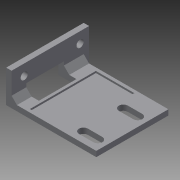
# Autodesk Inventor part: bart z endstop bracket v9
Saved by Autodesk Inventor 2014 SP1 (Build 180222100, 222)
## iProperties
Created: 2015-07-08
Part Number: bart z endstop bracket v9
Material: Generic
Document SubType Name: Modeling
Designer: Mon
Density: 1 g/cm^3
Appearance: Default
Author: Mon
Autodesk Inventor part; units mm, degrees
ref_plane "YZ Plane" through (0, 0, 0) normal (1, 0, 0) x (0, 1, 0)
ref_plane "XZ Plane" through (0, 0, 0) normal (0, 1, 0) x (-1, 0, 0)
ref_plane "XY Plane" through (0, 0, 0) normal (0, 0, 1) x (1, 0, 0)
sketch "Sketch1" plane through (0, 0, 0) normal (0, 0, 1) x (1, 0, 0)
  line L0 (0, 0) -> (50, 0)
  line L1 (50, 0) -> (50, -40)
  line L2 (50, -40) -> (0, -40)
  line L3 (0, -40) -> (0, 0)
  dimension "d0" = 50
  dimension "d1" = 40
  constraints: 8 end point, 2 parallel, 1 horizontal, 1 perpendicular
  measures "d0" distance of L1.end L2.end
  measures "d1" distance of L0.end L1.end
extrude "Extrusion1" add sketch "Sketch1" along normal blind 3
sketch "Sketch2" plane through (0, 0, 3) normal (0, 0, 1) x (1, 0, 0)
  line L0 (0, -40) -> (50, -40) projected
  line L1 (0, 0) -> (3, 0)
  line L2 (3, 0) -> (3, -40)
  line L3 (3, -40) -> (0, -40)
  line L4 (0, -40) -> (0, 0)
  dimension "d4" = 3
  constraints: 8 end point, 2 parallel, 1 horizontal, 1 perpendicular, 1 point on line
  measures "d4" distance of L2.end L3.end
extrude "Extrusion2" add sketch "Sketch2" along normal blind 15
sketch "Sketch3" plane through (0, 0, 0) normal (0, 1, 0) x (1, 0, 0)
  line L0 (0, 0) -> (3, 0)
  line L1 (3, 0) -> (3, -18)
  line L2 (3, -18) -> (0, -18)
  line L3 (0, -18) -> (0, 0)
  constraints: 8 end point, 2 parallel, 1 horizontal, 1 perpendicular
extrude "Extrusion3" add sketch "Sketch3" along normal blind 3
sketch "Sketch4" plane through (0, 0, 0) normal (0, 0, -1) x (-1, 0, 0)
  line L0 (0, -40) -> (0, 3) projected
  line L1 (-3, 0) -> (-3, 3) projected
  line L2 (-3, 0) -> (-3, -11)
  line L3 (0, -11) -> (-10, -11)
  line L4 (-10, -11) -> (-10, -31.8493)
  line L5 (-10, -31.8493) -> (0, -31.8493)
  point P0 (0, 0)
  dimension "d9" = 11
  dimension "d10" = 10
  constraints: 8 end point, 2 perpendicular, 2 point on line, 1 collinear, 1 parallel
  measures "d9" distance of L1.start L2.end
  measures "d10" distance of L3.start L3.end
extrude "Extrusion4" cut sketch "Sketch4" against normal blind 8
sketch "Sketch6" plane through (0, -40, 0) normal (-1, 0, 0) x (0, 0, 1)
  circle A0 centre (12, 38) radius 2
  point P0 (0, 40)
  dimension "d17" = 4
  constraints: 1 centre point
  measures "d17" diameter of A0
extrude "Extrusion6" cut sketch "Sketch6" against normal through all
sketch "Sketch7" plane through (0, -40, 0) normal (-1, 0, 0) x (0, 0, 1)
  circle A0 centre (12, 7) radius 2
  point P0 (0, 40)
  dimension "d21" = 4
  constraints: 1 centre point
  measures "d21" diameter of A0
extrude "Extrusion7" cut sketch "Sketch7" against normal through all
sketch "Sketch8" plane through (0, 0, 0) normal (0, 0, -1) x (-1, 0, 0)
  line L0 (-45, -12) -> (-37, -12) construction
  line L1 (-45, -14.5) -> (-37, -14.5)
  line L2 (-37, -9.5) -> (-45, -9.5)
  arc A0 (-45, -9.5) -> (-45, -14.5) centre (-45, -12) ccw
  arc A1 (-37, -14.5) -> (-37, -9.5) centre (-37, -12) ccw
  point P0 (0, 0)
  point P1 (-41, -12)
  dimension "d27" = 8
  dimension "d28" = 5
  constraints: 8 end point, 4 point on circle, 4 tangent, 2 centre point, 1 midpoint, 1 parallel
  measures "d27" distance of L0.start L0.end
  measures "d28" diameter of A1
extrude "Extrusion8" cut sketch "Sketch8" against normal through all
sketch "Sketch9" plane through (0, 0, 0) normal (0, 0, -1) x (-1, 0, 0)
  line L0 (-37, -14.5) -> (-45, -14.5) projected
  line L1 (-45, -34.1343) -> (-37, -34.1343) construction
  line L2 (-45, -36.6343) -> (-37, -36.6343)
  line L3 (-37, -31.6343) -> (-45, -31.6343)
  arc A0 (-45, -31.6343) -> (-45, -36.6343) centre (-45, -34.1343) ccw
  arc A1 (-37, -36.6343) -> (-37, -31.6343) centre (-37, -34.1343) ccw
  point P0 (0, 0)
  point P1 (-41, -34.1343)
  dimension "d31" = 8
  dimension "d32" = 5
  constraints: 8 end point, 4 point on circle, 4 tangent, 2 centre point, 2 parallel, 1 midpoint
  measures "d31" distance of L1.start L1.end
  measures "d32" diameter of A1
extrude "Extrusion9" cut sketch "Sketch9" against normal through all
sketch "Sketch10" plane through (0, 0, 3) normal (0, 0, 1) x (1, 0, 0)
  line L0 (11.4775, -1.7089) -> (32.8001, -1.7089)
  line L1 (32.8001, -1.7089) -> (32.8001, -38.2911)
  line L2 (32.8001, -38.2911) -> (11.4775, -38.2911)
  line L3 (11.4775, -38.2911) -> (11.4775, -1.7089)
  point P0 (0, 0)
  constraints: 8 end point, 2 parallel, 1 horizontal, 1 perpendicular
extrude "Extrusion10" cut sketch "Sketch10" against normal blind 1
chamfer "Chamfer1" distance 3 angle 45 1 edges at (3, -35.9246, 3)
chamfer "Chamfer2" distance 3 angle 45 1 edges at (3, -5.5, 3)
body "Solid1"
